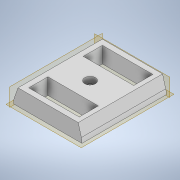
# Autodesk Inventor part: tripodInlay
Saved by Autodesk Inventor 2021 (Build 250183000, 183)
## iProperties
Created: 2020-07-08
Part Number: tripodInlay
Material: Generisch
Document SubType Name: Modeling
Designer: marvi
Density: 1 g/cm^3
Appearance: Vorgabe
Author: marvi
Autodesk Inventor part; units mm, degrees
sketch "Skizze1" plane through (0, 0, 0) normal (0, 0, 1) x (1, 0, 0)
  line L0 (0, 0) -> (42.19, 0)
  line L1 (2.6, 0) -> (2.6, 10)
  line L2 (39.89, 0) -> (39.89, 10)
  line L3 (2.6, 10) -> (39.89, 10)
  line L4 (0, 0) -> (-0.1073, 1.8337) construction
  spline S0 degree 3 poles (0, 0) (-0.1073, 1.8337) (0.0261, 2.9533) (0.334, 3.6563) knots 1 1 1 1 1.405888 1.405888 1.405888 1.405888
  line L5 (42.19, 0) -> (42.2285, 1.1988) construction
  spline S1 degree 3 poles (42.19, 0) (42.2285, 1.1988) (42.1183, 2.1671) (41.8072, 2.9533) knots 1 1 1 1 1.467938 1.467938 1.467938 1.467938
  line L6 (2.6, 10) -> (0.334, 3.6563)
  line L7 (-0.1073, 1.8337) -> (0.0261, 2.9533) construction
  line L8 (0.0261, 2.9533) -> (0.334, 3.6563) construction
  line L9 (39.89, 10) -> (41.8072, 2.9533)
  line L10 (42.2285, 1.1988) -> (42.1183, 2.1671) construction
  line L11 (42.1183, 2.1671) -> (41.8072, 2.9533) construction
  point P0 (39.89, 5)
  point P1 (2.6, 5)
  dimension "d0" = 42.19
  dimension "d1" = 2.6
  dimension "d2" = 10
  dimension "d3" = 2.3
  constraints: 12 end point, 2 horizontal, 2 midpoint, 2 point on line, 2 vertical, 6 other
  measures "d0" distance of L0.start L0.end
  measures "d1" distance from line of L1 L0.start
  measures "d2" distance of L1.start L1.end
  measures "d3" distance from line of L2 L0.end
extrude "Extrusion1" add sketch "Skizze1" along normal blind 52.21
sketch "Skizze3" plane through (0, 0, 0) normal (0, -1, 0) x (1, 0, 0)
  line L0 (0, 0) -> (42.19, 0) projected
  line L1 (0, 52.21) -> (42.19, 52.21) projected
  line L2 (42.19, 0) -> (42.19, 52.21) projected
  line L3 (0, 0) -> (0, 52.21) projected
  point P0 (21.095, 26.105)
hole "Bohrung2" at (21.095, 0, 26.105) direction (0, 1, 0) diameter 6.6 depth 10 counterbore diameter 15 counterbore depth 6
sketch "Skizze4" plane through (2.6, 10, 0) normal (0, 1, 0) x (1, 0, 0)
  line L0 (3.3345, -3.2969) -> (34.5895, -3.2969)
  line L1 (34.5895, -3.2969) -> (34.5895, -15.1659)
  line L2 (34.5895, -15.1659) -> (3.3345, -15.1659)
  line L3 (3.3345, -15.1659) -> (3.3345, -3.2969)
  circle A0 centre (18.495, -26.105) radius 3.3 projected
  line L4 (37.29, 0) -> (0, 0) projected
  line L5 (0, 0) -> (0, -52.21) projected
  line L6 (37.29, -52.21) -> (0, -52.21) projected
  line L7 (37.29, 0) -> (37.29, -52.21) projected
  line L8 (18.495, -26.105) -> (-9.8533, -26.105)
  line L9 (3.3345, -48.9131) -> (34.5895, -48.9131)
  line L10 (34.5895, -48.9131) -> (34.5895, -37.0441)
  line L11 (34.5895, -37.0441) -> (3.3345, -37.0441)
  line L12 (3.3345, -37.0441) -> (3.3345, -48.9131)
  point P0 (-2.6, 0)
  constraints: 18 end point, 4 symmetric about line, 2 horizontal, 2 parallel, 1 perpendicular
extrude "Extrusion2" cut sketch "Skizze4" against normal through all contours L0 L1 L2 L3 | L12 L11 L10 L9
